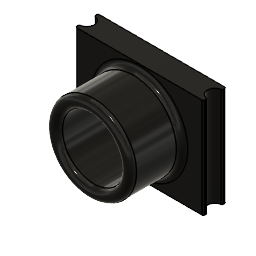
Motor Holder v1 (Autodesk Fusion 360 design; units mm, degrees)
Autodesk Fusion 360 part; units mm, degrees
sketch "Sketch1" plane through (0, 0, 0) normal (0, 1, 0) x (1, 0, 0)
  line L0 (22.5, 4) -> (-22.5, 4)
  line L1 (-22.5, 4) -> (-22.5, -4)
  line L2 (-22.5, -4) -> (22.5, -4)
  line L3 (22.5, -4) -> (22.5, 4)
  line L4 (22.5, 4) -> (-22.5, -4) construction
  line L5 (-22.5, 4) -> (22.5, -4) construction
  dimension "d1" = 45
  dimension "d2" = 8
  constraint horizontal L0
  constraint perpendicular L0 L1
  constraint parallel L0 L2
  constraint parallel L1 L3
  constraint coincident L4 origin
  constraint coincident L5 origin
  measures "d1" distance of L1.end L2.end
  measures "d2" distance of L0.end L1.end
extrude "Extrude1" add sketch "Sketch1" along normal blind 40
sketch "Sketch2" plane through (0, 0, 4) normal (0, 0, 1) x (1, 0, 0)
  line L0 (-22.5, 0) -> (22.5, 0)
  line L1 (22.5, 0) -> (22.5, 40)
  line L2 (22.5, 40) -> (-22.5, 40)
  line L3 (-22.5, 40) -> (-22.5, 0)
  line L4 (0, 40) -> (0, 0) construction
  line L5 (-22.5, 20) -> (22.5, 20) construction
  circle A0 centre (0, 20) radius 10
  circle A1 centre (0, 20) radius 7.5
  circle A2 centre (0, 20) radius 6.25
  circle A3 centre (0, 20) radius 3.75
  line L6 (0, 20) -> (0, 27.5)
  circle A4 centre (0, 27.5) radius 1.15
  line L7 (0, 20) -> (6.4952, 16.25)
  line L8 (0, 20) -> (7.5, 20) construction
  circle A5 centre (6.4952, 16.25) radius 1.15
  line L9 (0, 20) -> (-6.4952, 16.25)
  line L10 (0, 20) -> (7.5, 20) construction
  circle A6 centre (-6.4952, 16.25) radius 1.15
  dimension "d7" = 20
  dimension "d8" = 15
  dimension "d9" = 12.5
  dimension "d10" = 7.5
  dimension "d11" = 2.3
  dimension "d12" = 30
  dimension "d13" = 2.3
  dimension "d14" = 150
  dimension "d15" = 2.3
  constraint midpoint L2 L4.start
  constraint coincident L4.end origin
  constraint midpoint L3 L5.start
  constraint midpoint L1 L5.end
  constraint midpoint L5 A0.centre
  constraint concentric A0 A1
  constraint concentric A0 A2
  constraint concentric A1 A3
  constraint coincident A0.centre A1.centre
  constraint coincident A1 L6.end
  constraint coincident L4 L6.end
  constraint coincident L6.end A4.centre
  constraint horizontal L8
  constraint coincident L7.end A5.centre
  constraint horizontal L10
  constraint coincident L9.end A6.centre
  measures "d7" diameter of A0
  measures "d8" diameter of A1
  measures "d9" diameter of A2
  measures "d10" diameter of A3
  measures "d11" diameter of A4
  measures "d12" angle of L7 L8
  measures "d13" diameter of A5
  measures "d14" angle of L9 L10
  measures "d15" diameter of A6
extrude "Extrude2" cut sketch "Sketch2" against normal blind 4.3 contours A0 | A1 A2 L6 A4 L7 A5 | A1 L6 A4 | A1 A4 | A1 A5 | A1 L7 A5 | A1 L6 A4 | A1 A2 L6 A4 L9 A6 | A1 L7 A5 | A1 A2 L7 A5 L9 A6 | A1 L9 A6 | A1 A6 | A1 L9 A6
extrude "Extrude3" cut sketch "Sketch2" against normal blind 4.3 contours A2 A3 L6 L9 | A2 A3 L6 L7 | A2 A3 L7 L9 | A3 L6 L9 | A3 L6 L7 | A3 L7 L9
extrude "Extrude4" cut sketch "Sketch2" against normal blind 5.8 contours A2 A3 L6 L9 | A2 A3 L6 L7 | A2 A3 L7 L9 | A3 L6 L9 | A3 L6 L7 | A3 L7 L9
extrude "Extrude5" cut sketch "Sketch2" against normal blind 8 contours A3 L6 L9 | A3 L6 L7 | A3 L7 L9
extrude "Extrude6" cut sketch "Sketch2" against normal blind 8 contours A1 L6 A4 | A1 A4 | A1 A5 | A1 L7 A5 | A1 L6 A4 | A1 L7 A5 | A1 L9 A6 | A1 A6 | A1 L9 A6
sketch "Sketch3" plane through (0, 0, -4) normal (0, 0, -1) x (-1, 0, 0)
  circle A0 centre (0, 27.5) radius 1.15
  circle A1 centre (6.4952, 16.25) radius 1.15
  circle A2 centre (-6.4952, 16.25) radius 1.15
  circle A3 centre (0, 20) radius 3.75
  line L0 (-22.5, 0) -> (22.5, 0)
  line L1 (22.5, 40) -> (-22.5, 40)
  circle A4 centre (0, 27.5) radius 2.25
  circle A5 centre (-6.4952, 16.25) radius 2.25
  circle A6 centre (6.4952, 16.25) radius 2.25
  line L2 (22.5, 0) -> (22.5, 40)
  line L3 (-22.5, 40) -> (-22.5, 0)
  dimension "d26" = 4.5
  dimension "d27" = 4.5
  dimension "d28" = 4.5
  constraint concentric A0 A4
  constraint concentric A2 A5
  constraint concentric A1 A6
  measures "d26" diameter of A4
  measures "d27" diameter of A5
  measures "d28" diameter of A6
extrude "Extrude7" cut sketch "Sketch3" against normal blind 2 contours A4 | A5 | A6
sketch "Sketch4" plane through (0, 0, 4) normal (0, 0, 1) x (1, 0, 0)
  line L0 (-22.5, 0) -> (22.5, 0)
  line L1 (22.5, 0) -> (22.5, 40)
  line L2 (22.5, 40) -> (-22.5, 40)
  line L3 (-22.5, 40) -> (-22.5, 0)
  circle A0 centre (0, 20) radius 10
  circle A1 centre (0, 20) radius 11
  circle A2 centre (0, 20) radius 15
  dimension "d31" = 22
  dimension "d32" = 30
  constraint concentric A0 A1
  constraint concentric A1 A2
  measures "d31" diameter of A1
  measures "d32" diameter of A2
extrude "Extrude8" add sketch "Sketch4" along normal blind 20 contours A2
extrude "Extrude13" cut 1 faces at (7.5, 40, 1.3333) along direction (0, -1, 0) blind 2.5
extrude "Extrude14" cut 1 faces at (7.5, 0, 1.3333) along direction (0, 1, 0) blind 2.5
sketch "Sketch5" plane through (0, 0, -4) normal (0, 0, -1) x (-1, 0, 0)
  line L0 (-22.5, 2.5) -> (22.5, 2.5)
  line L1 (22.5, 37.5) -> (-22.5, 37.5)
  circle A0 centre (0, 20) radius 3.75
  circle A1 centre (6.4952, 16.25) radius 2.25
  circle A2 centre (0, 27.5) radius 2.25
  circle A3 centre (-6.4952, 16.25) radius 2.25
  circle A4 centre (0, 20) radius 14.5
  circle A5 centre (0, 20) radius 19.5
  line L2 (22.5, 2.5) -> (22.5, 37.5)
  line L3 (-22.5, 37.5) -> (-22.5, 2.5)
  dimension "d55" = 29
  dimension "d56" = 39
  constraint concentric A0 A4
  constraint concentric A4 A5
  measures "d55" diameter of A4
  measures "d56" diameter of A5
sketch "Sketch6" plane through (0, 0, -4) normal (0, 0, -1) x (-1, 0, 0)
  line L0 (-22.5, 2.5) -> (22.5, 2.5)
  line L1 (22.5, 37.5) -> (-22.5, 37.5)
  circle A0 centre (0, 20) radius 3.75
  circle A1 centre (6.4952, 16.25) radius 2.25
  circle A2 centre (0, 27.5) radius 2.25
  circle A3 centre (-6.4952, 16.25) radius 2.25
  circle A4 centre (0, 20) radius 11.5
  circle A5 centre (0, 20) radius 10
  line L2 (22.5, 2.5) -> (22.5, 37.5)
  line L3 (-22.5, 37.5) -> (-22.5, 2.5)
  dimension "d61" = 23
  dimension "d62" = 20
  constraint concentric A0 A4
  constraint concentric A0 A5
  measures "d61" diameter of A4
  measures "d62" diameter of A5
extrude "Extrude17" cut sketch "Sketch6" against normal blind 2 contours L0 L1 L2 L3
fillet "Fillet8" radius 1 2 edges at (10.7218, 15.8414, -2) (10.7218, 15.8414, -4)
sketch "Sketch7" plane through (0, 0, 4) normal (0, 0, 1) x (1, 0, 0)
  line L0 (-22.5, 2.5) -> (22.5, 2.5)
  line L1 (22.5, 37.5) -> (-22.5, 37.5)
  line L2 (-22.5, 37.5) -> (-22.5, 2.5)
  line L3 (-22.5, 37.5) -> (22.5, 37.5)
  line L4 (22.5, 37.5) -> (22.5, 2.5)
  line L5 (22.5, 2.5) -> (-22.5, 2.5)
  line L6 (-22.5, 2.5) -> (-22.5, 37.5)
  circle A0 centre (0, 20) radius 10
  circle A1 centre (0, 20) radius 15
  circle A2 centre (0, 20) radius 15
  line L7 (22.5, 2.5) -> (22.5, 37.5)
  dimension "d73" = 45
  dimension "d74" = 35
  dimension "d75" = 20
  dimension "d76" = 30
  constraint horizontal L3
  constraint vertical L4
  constraint horizontal L5
  constraint vertical L6
  constraint coincident L1.end L2.start
  constraint concentric A0 A1
  measures "d73" distance of L1.end L1.start
  measures "d74" distance of L1.end L0.start
  measures "d75" diameter of A0
  measures "d76" diameter of A1
extrude "Extrude18" add sketch "Sketch7" along normal blind 2 contours L0 L1 L2 L3 L4 L5 L6 L7
fillet "Fillet9" radius 2 3 edges at (-13.9849, 14.5758, 6) (-13.9849, 14.5758, 24) (-10.2556, 23.9778, 24)
sketch "Sketch8" plane through (0, 37.5, 0) normal (0, 1, 0) x (-1, 0, 0)
  line L0 (-22.5, -2) -> (22.5, -2)
  line L1 (22.5, -2) -> (22.5, 6)
  line L2 (22.5, 6) -> (-22.5, 6)
  line L3 (-22.5, 6) -> (-22.5, -2)
  circle A0 centre (-22.5, 2) radius 2.6
  circle A1 centre (22.5, 2) radius 2.65
  dimension "d81" = 5.2
  dimension "d82" = 5.3
  constraint midpoint L3 A0.centre
  constraint midpoint L1 A1.centre
  measures "d81" diameter of A0
  measures "d82" diameter of A1
extrude "Extrude19" cut sketch "Sketch8" against normal blind 35 contours L3 A0 | L3 A0 | L1 A1 | L1 A1
fillet "Fillet10" radius 0.5 8 edges at (-22.5, 20, -2) (-22.5, 20, 4.65) (22.5, 20, -2) (22.5, 20, 4.6) (22.5, 20, 6) (22.5, 20, -0.6) (-22.5, 20, 6) (-22.5, 20, -0.65)
equation "d14 = 180 deg - 30 deg"
equation "d81 = ( 2.6 * 2 ) * 1 mm"
